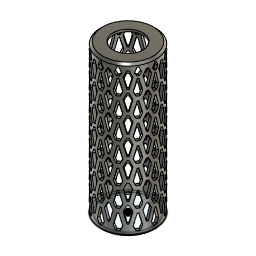
led-lamp-shade (Autodesk Fusion 360 design; units mm, degrees)
Autodesk Fusion 360 part; units mm, degrees
sketch "Sketch1" plane through (0, 0, 0) normal (0, 0, 1) x (1, 0, 0)
  circle A0 centre (0, 0) radius 39.5
  circle A1 centre (0, 0) radius 35.5
  dimension "d1" = 79
  dimension "d2" = 71
  constraint coincident A0.centre A1.centre
  measures "d1" diameter of A0
  measures "d2" diameter of A1
extrude "Extrude12" add sketch "Sketch1" along normal blind 210
sketch "Sketch16" plane through (0, 0, 0) normal (0, 0, 1) x (1, 0, 0)
  circle A0 centre (0, 0) radius 35.625
  circle A1 centre (0, 0) radius 37.125
  dimension "d132" = 71.25
  dimension "d133" = 1.5
  constraint coincident A0.centre A1.centre
  constraint concentric A0 A1
  measures "d132" diameter of A0
  measures "d133" distance of A0 A1
extrude "Extrude15" add sketch "Sketch16" against normal blind 3
ref_plane "WorkPlane2" through (0, -40, 0) normal (0, 1, 0) x (0, 0, 1)
sketch "Sketch4" plane through (0, -40, 0) normal (0, 1, 0) x (1, 0, 0)
  line L0 (-6.6987, -4) -> (0, -29)
  line L1 (0, -29) -> (6.6987, -4)
  line L2 (6.6987, -4) -> (-6.6987, -4)
  line L3 (0, 0) -> (0, -4)
  line L4 (0.8038, -26) -> (-0.8038, -26)
  line L5 (2.1987, -4) -> (5.0566, -10.1286)
  line L6 (-2.1987, -4) -> (-5.0566, -10.1286)
  dimension "d11" = 75
  dimension "d18" = 4
  dimension "d46" = 3
  dimension "d77" = 25
  dimension "d93" = 4.5
  dimension "d94" = 4.5
  dimension "d95" = 40
  dimension "d96" = 40
  constraint horizontal L2
  constraint equal L0 L1
  constraint coincident L3.start origin
  constraint midpoint L2 L3.end
  constraint vertical L3
  constraint horizontal L4
  constraint coincident L1 L4.start
  constraint coincident L0 L4.end
  constraint coincident L2 L6.start
  constraint coincident L0 L6.end
  constraint coincident L2 L5.start
  constraint coincident L1 L5.end
  measures "d11" angle of L1 L2
  measures "d18" distance of L3.start L2
  measures "d46" distance of L0.end L4
  measures "d77" distance of L0.end L2
  measures "d93" distance of L1.end L5.start
  measures "d94" distance of L0.start L6.start
  measures "d95" angle of L0 L6
  measures "d96" angle of L1 L5
extrude "Extrude13" cut sketch "Sketch4" along normal up to surface contours L0 L1 L2 L4 L5 L6 end surface at (35.3236, -3.5347, 140)
pattern_circular "C-Pattern3" count 12 over 360 about axis through (0, 0, 1.75) along (0, 0, 1) of "Extrude13"
pattern_linear "R-Pattern4" count 7 spacing 28 along (0, 0, 1) of "Extrude13", "C-Pattern3"
ref_plane "WorkPlane7" through (0, 0, 12.125) normal (-0.258819, 0.965926, 0) x (0, 0, 1)
ref_plane "WorkPlane8" through (12.941, -48.2963, 12.125) normal (-0.258819, 0.965926, 0) x (0, 0, 1)
sketch "Sketch15" plane through (12.941, -48.2963, 12.125) normal (-0.258819, 0.965926, 0) x (0, 0, 1)
  line L0 (23.875, -1.2693) -> (16, -5)
  line L1 (23.875, -7.0588) -> (23.875, 7.0588)
  line L2 (0.875, -1.0458) -> (0.875, 1.0458)
  line L3 (-3.125, 0) -> (23.875, -7.0588)
  line L4 (23.875, 1.2693) -> (16, 5)
  line L5 (23.875, 7.0588) -> (-3.125, 0)
  line L6 (-3.125, 0) -> (-12.125, 0)
  point P0 (-12.125, 0)
  dimension "d117" = 4
  dimension "d121" = 40
  dimension "d122" = 40
  dimension "d123" = 9
  dimension "d137" = 27
  constraint equal L3 L5
  constraint coincident L2.start L3
  constraint coincident L2.end L5
  constraint coincident L4.start L1
  constraint coincident L4.end L5
  constraint coincident L0.start L1
  constraint coincident L0.end L3
  constraint coincident P0 L6.end
  constraint horizontal L6
  constraint perpendicular L1 L6
  constraint perpendicular L2 L6
  constraint equal L0 L4
  measures "d117" distance of L3.start L2
  measures "d121" angle of L4 L5
  measures "d122" angle of L0 L3
  measures "d123" distance of L3.start P0
  measures "d137" distance of L3.start L1
extrude "Extrude14" cut sketch "Sketch15" along normal up to surface contours L0 L1 L2 L3 L4 L5 end surface at (-8.7599, -34.4022, 62.7524)
pattern_circular "C-Pattern4" count 12 over 360 about axis through (0, 0, 1.75) along (0, 0, 1) of "Extrude14"
pattern_linear "R-Pattern5" count 7 spacing 28 along (0, 0, 1) of "Extrude14", "C-Pattern4"
sketch "Sketch18" plane through (0, 0, 0) normal (0, 1, 0) x (1, 0, 0)
  line L0 (-4, -201) -> (-1, -208)
  line L1 (-1, -197) -> (-4, -201)
  line L2 (-4, -201) -> (4, -201)
  line L3 (-0.8038, -194) -> (0.8038, -194)
  line L4 (-1, -208) -> (1, -208)
  line L5 (1, -208) -> (4, -201)
  line L6 (-1, -197) -> (1, -197)
  line L7 (1, -197) -> (4, -201)
  line L8 (0, -197) -> (0, -194)
  dimension "d139" = 11
  dimension "d140" = 8
  dimension "d141" = 2
  dimension "d142" = 2
  dimension "d143" = 7
  dimension "d144" = 3
  constraint horizontal L2
  constraint horizontal L4
  constraint midpoint L6 L8.start
  constraint midpoint L3 L8.end
  constraint perpendicular L3 L8
  constraint perpendicular L6 L8
  constraint equal L0 L5
  constraint equal L1 L7
  measures "d139" distance of L0.end L1.start
  measures "d140" horizontal distance of L0.start L2.end
  measures "d141" distance of L1.start L6.end
  measures "d142" distance of L0.end L4.end
  measures "d143" distance of L2 L4
  measures "d144" distance of L8.start L8.end
extrude "Extrude16" cut sketch "Sketch18" along normal up to surface end surface at (39.4149, -2.5914, 203.3405)
pattern_circular "C-Pattern5" count 12 over 360 about axis through (0, 0, 1.75) along (0, 0, 1) of "Extrude16"
sketch "Sketch19" plane through (0, 0, 210) normal (0, 0, 1) x (-1, 0, 0)
  circle A0 centre (0, 0) radius 35.5
  circle A1 centre (0, 0) radius 39.5
  circle A2 centre (0, 0) radius 21.5
  dimension "d149" = 43
  constraint coincident A0.centre A1.centre
  measures "d149" diameter of A2
extrude "Extrude17" add sketch "Sketch19" along normal blind 3 contours A0 | A1
chamfer "Chamfer3" distance 3 angle 45 1 edges at (36.8269, 14.2838, 213)
